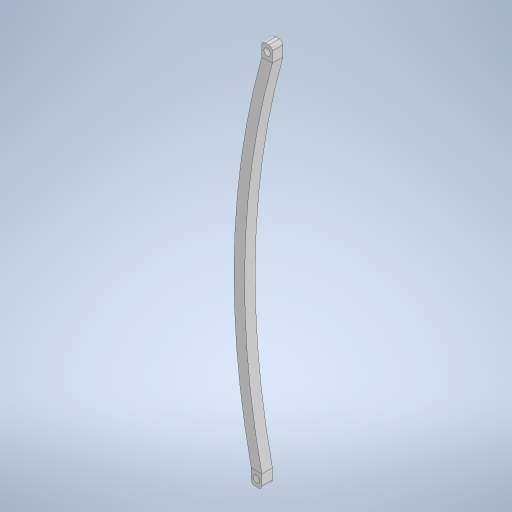
# Autodesk Inventor part: ferris_wheel_outer_ring
Saved by Autodesk Inventor 2023 (Build 270158000, 158)
## iProperties
Created: 2025-10-20
Part Number: ferris_wheel_outer_ring
Material: Generic
Document SubType Name: Modeling
Designer: Justin Pascual
Density: 1 g/cm^3
Appearance: Default
Author: Justin Pascual
Autodesk Inventor part; units mm, degrees
ref_plane "YZ Plane" through (0, 0, 0) normal (1, 0, 0) x (0, 1, 0)
ref_plane "XY Plane" through (0, 0, 0) normal (0, 0, 1) x (1, 0, 0)
sketch "Sketch2" plane through (0, 0, 0) normal (0, 1, 0) x (-1, 0, 0)
  line L0 (0, 0) -> (-3.81, 0)
  line L1 (-3.81, 0) -> (-3.81, -3.81)
  line L2 (-3.81, -3.81) -> (0, -3.81)
  line L3 (0, -3.81) -> (0, 0)
  dimension "d4" = 3.81
  dimension "d5" = 3.81
  constraints: 8 end point, 2 parallel, 1 horizontal, 1 perpendicular
  measures "d4" distance of L2.end L1.end
  measures "d5" distance of L1.end L0.end
ref_plane "Work Plane1" through (0, 131.826, 0) normal (0, 1, 0) x (-1, 0, 0)
sketch "Sketch3" plane through (0, 131.826, 0) normal (0, 1, 0) x (-1, 0, 0)
  line L0 (-3.81, -3.81) -> (0, -3.81) projected
  line L1 (0, -3.81) -> (0, 0) construction
  line L2 (-3.81, 0) -> (-3.81, -3.81) construction
  line L3 (0, 0) -> (-3.81, 0) construction
  line L4 (-3.81, -3.81) -> (0, -3.81)
  line L5 (0, -3.81) -> (0, -7.62)
  line L6 (0, -7.62) -> (-3.81, -7.62)
  line L7 (-3.81, -7.62) -> (-3.81, -3.81)
  dimension "d7" = 3.81
  dimension "d8" = 3.81
  constraints: 8 end point, 2 parallel, 1 horizontal, 1 perpendicular
  measures "d7" distance of L5.end L6.end
  measures "d8" distance of L4.end L5.end
ref_plane "Work Plane2" through (3.81, 0, -3.81) normal (0, -0.0288897, -0.9995826) x (-1, 0, 0)
ref_plane "Work Plane3" through (0, 2.54, 0) normal (0, 1, 0) x (-1, 0, 0)
sketch "Sketch5" plane through (0, 2.54, 0) normal (0, 1, 0) x (-1, 0, 0)
  line L0 (0, 0) -> (-3.81, 0) construction
  line L1 (0, 0) -> (-3.81, 0) projected
  line L2 (-3.81, 0) -> (-3.81, -3.81) projected
  line L3 (-3.81, -3.81) -> (0, -3.81) projected
  line L4 (0, -3.81) -> (0, 0) projected
ref_plane "Work Plane4" through (0, 129.286, 0) normal (0, 1, 0) x (-1, 0, 0)
sketch "Sketch6" plane through (0, 129.286, 0) normal (0, 1, 0) x (-1, 0, 0)
  line L0 (0, -7.62) -> (-3.81, -7.62) projected
  line L1 (0, -3.81) -> (0, -7.62) projected
  line L2 (-3.81, -3.81) -> (0, -3.81) projected
  line L3 (-3.81, -7.62) -> (-3.81, -3.81) projected
  point P0 (0, 0)
ref_plane "Work Plane5" through (0, 129.286, -7.62) normal (0, -0.0300465, -0.9995485) x (1, 0, 0)
sketch "Sketch8" plane through (0, 129.286, -7.62) normal (0, -0.0300465, -0.9995485) x (1, 0, 0)
  circle A0 centre (245.9598, 63.4016) radius 254 construction
  arc A1 (0, 126.8033) -> (0, 0) centre (245.9598, 63.4016) ccw
  point P0 (0, 129.4566)
  dimension "d13" = 508
  constraints: 4 point on circle, 2 centre point, 1 concentric
  measures "d13" diameter of A0
sweep "Sweep1" add profiles "Sketch5" path "Sketch8" keep normal constant yes
extrude "Extrusion2" add sketch "Sketch3" along normal mid plane 5.08
extrude "Extrusion3" add sketch "Sketch2" along normal mid plane 5.08
sketch "Sketch10" plane through (0, 134.366, -3.81) normal (0, 0, 1) x (1, 0, 0)
  line L0 (0, 0) -> (3.81, 0) projected
  point P0 (0, -134.366)
  point P1 (1.905, -2.54)
  dimension "d20" = 2.54
  measures "d20" distance from line of L0 point (1.905, -2.54)
hole "Hole1" at (1.905, 131.826, -3.81) direction (0, 0, -1) diameter 2.4384 end through all
fillet "Fillet1" radius 1.27 2 edges at (0, 134.366, -5.715) (3.81, 134.366, -5.715)
sketch "Sketch11" plane through (0, 2.54, 0) normal (0, 0, 1) x (1, 0, 0)
  line L0 (3.81, -5.08) -> (0, -5.08) projected
  point P0 (0, -2.54)
  point P1 (1.905, -2.54)
  dimension "d29" = 2.54
  measures "d29" distance from line of L0 point (1.905, -2.54)
hole "Hole2" at (1.905, 0, 0) direction (0, 0, -1) diameter 2.4384 end through all
fillet "Fillet2" radius 1.27 2 edges at (0, -2.54, -1.905) (3.81, -2.54, -1.905)
body "Solid2"
